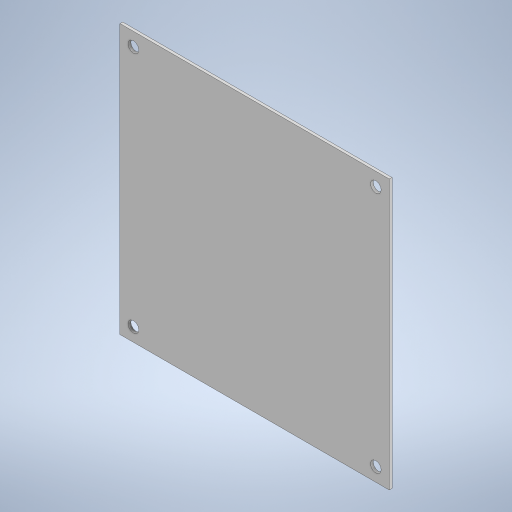
# Autodesk Inventor part: plate
Saved by Autodesk Inventor 2023 (Build 270158000, 158)
## iProperties
Created: 2022-09-29
Part Number: plate
Material: Generic
Document SubType Name: Sheet Metal
Designer: earls
Density: 1 g/cm^3
Sheet Metal Rule: Default_mm
Appearance: Default
Author: earls
Autodesk Inventor part; units mm, degrees
ref_plane "YZ Plane" through (0, 0, 0) normal (1, 0, 0) x (0, 1, 0)
ref_plane "XZ Plane" through (0, 0, 0) normal (0, 1, 0) x (-1, 0, 0)
ref_plane "XY Plane" through (0, 0, 0) normal (0, 0, 1) x (1, 0, 0)
sketch "Sketch1" plane through (0, 0, 0) normal (0, 0, 1) x (1, 0, 0)
  line L0 (-130.9665, 63.5108) -> (69.0335, 63.5108)
  line L1 (69.0335, 63.5108) -> (69.0335, -136.4892)
  line L2 (69.0335, -136.4892) -> (-130.9665, -136.4892)
  line L3 (-130.9665, -136.4892) -> (-130.9665, 63.5108)
  circle A0 centre (-120.9665, 53.5108) radius 4
  line L4 (-30.9665, 63.5108) -> (-30.9665, 23.3683)
  line L5 (-130.9665, -36.4892) -> (-82.7476, -36.4892)
  circle A1 centre (59.0335, 53.5108) radius 4
  circle A2 centre (-120.9665, -126.4892) radius 4
  circle A3 centre (59.0335, -126.4892) radius 4
  point P0 (0, 0)
  dimension "d0" = 200
  dimension "d1" = 200
  dimension "d2" = 8
  dimension "d3" = 10
  dimension "d4" = 10
  measures "d0" distance of L0.start L0.end
  measures "d1" distance of L0.end L1.end
  measures "d2" diameter of A0
  measures "d3" distance from line of A0.centre L0
  measures "d4" distance from line of A0.centre L3
extrude "Plate1" add sketch "Sketch1" along normal mid plane 2
equation "\"d5\" = Thickness"
equation "\"BendRadius\" = Thickness"
equation "\"BendReliefWidth\" = Thickness"
equation "\"BendReliefDepth\" = 0.5 * Thickness"
equation "\"CornerReliefSize\" = 4 * Thickness"
equation "\"MinimumRemnant\" = 2 * Thickness"
equation "\"TransitionRadius\" = BendRadius"
equation "\"JacobiRadiusSize\" = BendRadius"
equation "\"GapSize\" = Thickness"
equation "\"Thickness\" = 2"
body "Solid1"
